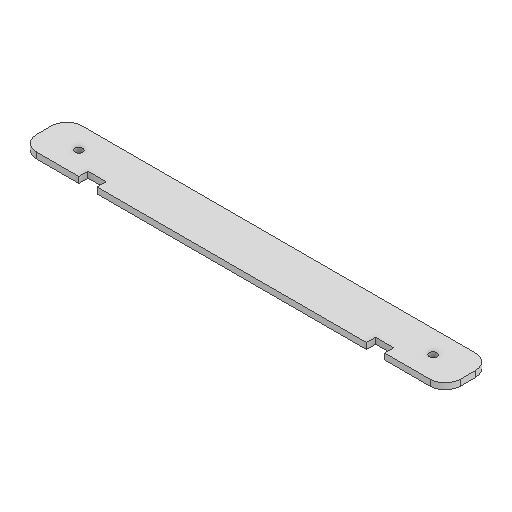
# Autodesk Inventor part: 3DP_PLA_Screw_Spacing_Test_Part
Saved by Autodesk Inventor 2025 (Build 290162010, 162A)
## iProperties
Created: 2024-10-10
Part Number: 3DP_PLA_Screw_Spacing_Test_Part
Material: Generic
Document SubType Name: Modeling
Designer: User
Density: 1 g/cm^3
Appearance: Default
Author: User
Autodesk Inventor part; units mm, degrees
ref_plane "YZ Plane" through (0, 0, 0) normal (1, 0, 0) x (0, 1, 0)
ref_plane "XZ Plane" through (0, 0, 0) normal (0, 1, 0) x (-1, 0, 0)
ref_plane "XY Plane" through (0, 0, 0) normal (0, 0, 1) x (1, 0, 0)
sketch "Sketch1" plane through (0, 0, 0) normal (0, 1, 0) x (-1, 0, 0)
  line L0 (70, 7.5) -> (-70, 7.5)
  line L1 (-70, 7.5) -> (-70, -7.5)
  line L2 (-70, -7.5) -> (70, -7.5)
  line L3 (70, -7.5) -> (70, 7.5)
  line L4 (51, 7.5) -> (51, 4.5)
  line L5 (51, 4.5) -> (45, 4.5)
  line L6 (45, 4.5) -> (45, 7.5)
  line L7 (-50, 7.5) -> (-50, 4.5)
  line L8 (-50, 4.5) -> (-44, 4.5)
  line L9 (-44, 4.5) -> (-44, 7.5)
  point P0 (0, 0)
  point P1 (58.5, 0)
  point P2 (-58.5, 0)
  point P3 (-70, 0)
  dimension "d0" = 117
  dimension "d1" = 58.5
  dimension "d2" = 140
  dimension "d3" = 70
  dimension "d4" = 7.5
  dimension "d5" = 15
  dimension "d6" = 7.5
  dimension "d7" = 6
  dimension "d8" = 3
  dimension "d9" = 7.5
  dimension "d10" = 6
  dimension "d11" = 3
  dimension "d12" = 101
  constraints: 20 end point, 5 perpendicular, 4 point on line, 2 parallel, 2 vertical, 1 horizontal, 1 horizontal alignment, 1 midpoint
  measures "d0" distance of point (-58.5, 0) point (58.5, 0)
  measures "d1" distance of point (0, 0) point (58.5, 0)
  measures "d2" distance from line of point (-70, 0) L3
  measures "d3" distance from line of L3 point (0, 0)
  measures "d4" distance from line of point (58.5, 0) L0
  measures "d5" distance between parallel lines of L2 L0
  measures "d6" distance from line of point (0, 0) L0
  measures "d7" distance between parallel lines of L6 L4
  measures "d8" distance between parallel lines of L0 L5
  measures "d9" distance from line of point (58.5, 0) L4
  measures "d10" distance between parallel lines of L7 L9
  measures "d11" distance between parallel lines of L8 L0
  measures "d12" distance between parallel lines of L4 L7
extrude "Extrusion1" add sketch "Sketch1" along normal blind 2 contours L3 L2 L1 L0 L7 L8 L9 L6 L5 L4
hole "Hole1" at (-58.5, 0, 0) at (58.5, 0, 0) direction (0, 1, 0) diameter 2.5 depth 6.5
fillet "Fillet1" radius 5 4 edges at (-70, 1, 7.5) (-70, 1, -7.5) (70, 1, 7.5) (70, 1, -7.5)
equation "\"d1\" = 0.5 * d0"
equation "\"d3\" = 0.5 * d2"
equation "\"d4\" = 0.5 * d5"
equation "\"d6\" = d4"
body "Solid1"
